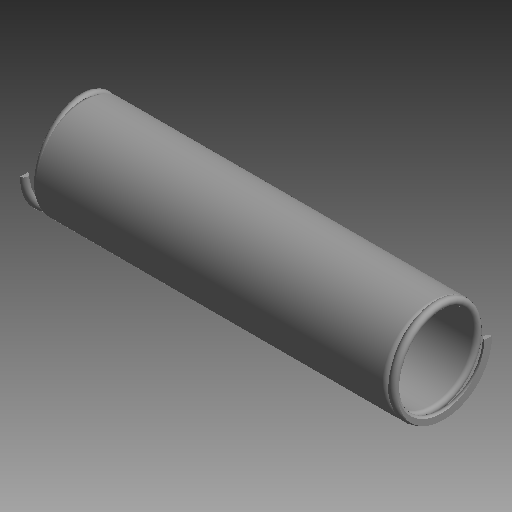
# Autodesk Inventor part: C206 (38)3d
Saved by Autodesk Inventor 2019 (Build 230136000, 136)
## iProperties
Category: PARTsolutions
Company: ACCURATE
Part Number: C206 (38)3d
Material: 一般
Catalog Web Link: www.cadenas.de
Description: C Standard-
Vendor: ACCURATE
Document SubType Name: Modeling
Designer: partserver
Manufacturer: ACCURATE
Mass: 0.84905 g
Surface Area: 22.0995 cm^2
Volume: 0.84905 cm^3
Density: 1 g/cm^3
Appearance: PSOLRGB-175-175-175
PSOL_IDENT_0: {$CADENAS_DATA\23d-libs\accurate\helical_compresion_spring\c_standard_3d.prj},163 {VTYP=3D},{NB=C206
PSOL_IDENT_1: (38)3d},{LINA=C206},{NN=C Standard},{DATE=27.01.2021 08:27:26},{GEOMDATE=03.04.2014 02:10:44},{VERS
PSOL_IDENT_2: ION=},{LINEID=1070},{WBVAR=H},{WBNUMERIC=H}  {NB=C206 (38)3d},{LINA=C206},{KT=DUMMY},{ORDER=C206},{H=
PSOL_IDENT_3: 38},{HF=38.0},{D=0.80},{OD=10.0},{P1=6.77},{H1=23.75},{P2=10.64},{H2=15.86},{K=0.481},{NT=11.50},{HS=
PSOL_IDENT_4: 9.20},{Q=10},{MAT=18-8 Stainless Steel Wire for Spring},{RID=G_1060},{STDRT=0.80},{DESCR=Creating of
PSOL_IDENT_5: the Templates - C Standard},{PAST=A},{REST=M},{VERS=6},{BL=2},{SC=1},{NTX=11},{L=38}
NB: C206 (38)3d
NN: C Standard
NT: 11.5
NBSYN: $ORDER. ($H.)3d
LINA: C206
CATALOG: Accurate Inc
ORDER: C206
H: 38
HF: 38
D: 0.8
OD: 10
P1: 6.77
H1: 23.75
P2: 10.64
H2: 15.86
K: 0.481
HS: 9.2
Q: 10
MAT: 18-8 Stainless Steel Wire for Spring
SUPPLIER: ACCURATE
ARTICLENO: C206 (38)3d
BOMINFO: C206
CREATOR: CADENAS GmbH
Title: C206
Author: Cadenas PARTsolutions
Autodesk Inventor part; units mm, degrees
ref_plane "YZ Plane" through (0, 0, 0) normal (1, 0, 0) x (0, 1, 0)
ref_plane "XZ Plane" through (0, 0, 0) normal (0, 1, 0) x (-1, 0, 0)
ref_plane "XY Plane" through (0, 0, 0) normal (0, 0, 1) x (1, 0, 0)
sketch "Sketch_14" plane through (0, 0, 0) normal (0, 0, 1) x (1, 0, 0)
  line L0 (-3.8, 0.4) -> (5.4, -0.4)
  circle A0 centre (0.4, -4.6) radius 0.4
  constraints: 2 end point, 1 centre point
revolve "Revolution1" add sketch "Sketch_14" angle 180 about axis through (-3.8, 0.4, 0) along (0.9962, -0.0866, 0)
sketch "Sketch_5" plane through (0, 0, 0) normal (0, 0, 1) x (1, 0, 0)
  line L0 (4.8, 0.2) -> (-4.4, -0.2)
  circle A0 centre (0, 4.6) radius 0.4
  constraints: 2 end point, 1 centre point
revolve "Revolution2" add sketch "Sketch_5" angle 180 about axis through (4.8, 0.2, 0) along (0.9991, 0.0434, 0)
sketch "Sketch_6" plane through (0, 0, 0) normal (0, 0, 1) x (1, 0, 0)
  line L0 (0, 0) -> (-0.8, 0)
  line L1 (-0.8, 0) -> (-0.8, 10)
  line L2 (-0.8, 10) -> (0, 10)
  line L3 (0, 10) -> (0, 0)
  line L4 (0, 0) -> (-0.8, 0)
  constraints: 10 end point
revolve "Revolution3" cut sketch "Sketch_6" angle 360 about axis through (0, 0, 0) along (1, 0, 0)
sketch "Sketch_30" plane through (0, 0, 0) normal (0, 0, 1) x (1, 0, 0)
  line L0 (38, 0) -> (-38, 0)
  arc A0 (1.19, 5) -> (1.19, 4.2) centre (1.19, 4.6) ccw
  line L1 (1.19, 4.2) -> (36.41, 4.2)
  arc A1 (36.41, 4.2) -> (36.41, 5) centre (36.41, 4.6) ccw
  line L2 (36.41, 5) -> (1.19, 5)
  constraints: 6 end point, 4 point on circle, 2 centre point
revolve "Revolution4" add sketch "Sketch_30" angle 360 about axis through (38, 0, 0) along (-1, 0, 0)
sketch "Sketch_18" plane through (0, 0, 0) normal (0, 0, 1) x (1, 0, 0)
  line L0 (41.6, -0.6) -> (32.4, 0.6)
  circle A0 centre (37.6, 4.6) radius 0.4
  constraints: 2 end point, 1 centre point
revolve "Revolution5" add sketch "Sketch_18" angle 180 about axis through (41.6, -0.6, 0) along (-0.9916, 0.1293, 0)
sketch "Sketch_19" plane through (0, 0, 0) normal (0, 0, 1) x (1, 0, 0)
  line L0 (42.4, 0.2) -> (33.2, -0.2)
  circle A0 centre (37.6, 4.6) radius 0.4
  constraints: 2 end point, 1 centre point
revolve "Revolution6" add sketch "Sketch_19" angle 180 about axis through (42.4, 0.2, 0) along (0.9991, 0.0434, 0)
sketch "Sketch_20" plane through (0, 0, 0) normal (0, 0, 1) x (1, 0, 0)
  line L0 (38.8, 0) -> (38, 0)
  line L1 (38, 0) -> (38, 10)
  line L2 (38, 10) -> (38.8, 10)
  line L3 (38.8, 10) -> (38.8, 0)
  line L4 (38.8, 0) -> (38, 0)
  constraints: 10 end point
revolve "Revolution7" cut sketch "Sketch_20" angle 360 about axis through (38.8, 0, 0) along (-1, 0, 0)
body "Solid1"
